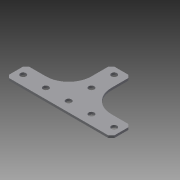
# Autodesk Inventor part: 3x5 T
Saved by Autodesk Inventor 2015 (Build 190159000, 159)
## iProperties
Created: 2015-01-29
Part Number: 3x5 T
Material: Generic
Document SubType Name: Sheet Metal
Designer: chappelled
Density: 1 g/cm^3
Appearance: Default
Sheet Metal Rule: Default
Author: chappelled
Autodesk Inventor part; units mm, degrees
ref_plane "YZ Plane" through (0, 0, 0) normal (1, 0, 0) x (0, 1, 0)
ref_plane "XZ Plane" through (0, 0, 0) normal (0, 1, 0) x (-1, 0, 0)
ref_plane "XY Plane" through (0, 0, 0) normal (0, 0, 1) x (1, 0, 0)
sketch "Sketch1" plane through (0, 0, 0) normal (0, 1, 0) x (-1, 0, 0)
  line L0 (-3.175, 0) -> (-19.05, 0)
  line L1 (-69.85, 50.8) -> (-69.85, 66.675)
  line L2 (-66.675, 69.85) -> (44.45, 69.85)
  line L3 (-66.675, 69.85) -> (-69.85, 66.675)
  line L4 (-22.225, 3.175) -> (-22.225, 22.225)
  line L5 (-47.625, 47.625) -> (-66.675, 47.625)
  arc A0 (-22.225, 22.225) -> (-47.625, 47.625) centre (-47.625, 22.225) ccw
  line L6 (-22.225, 3.175) -> (-19.05, 0)
  line L7 (-69.85, 50.8) -> (-66.675, 47.625)
  line L8 (0, 3.175) -> (0, 22.225)
  line L9 (25.4, 47.625) -> (44.45, 47.625)
  line L10 (47.625, 50.8) -> (47.625, 66.675)
  arc A1 (25.4, 47.625) -> (0, 22.225) centre (25.4, 22.225) ccw
  line L11 (44.45, 69.85) -> (47.625, 66.675)
  line L12 (44.45, 47.625) -> (47.625, 50.8)
  line L13 (-3.175, 0) -> (0, 3.175)
  point P0 (0, 0)
  point P1 (-69.85, 69.85)
  point P2 (-3.175, 0)
  point P3 (0, 0)
  point P4 (-22.225, 47.625)
  point P5 (-22.225, 0)
  point P6 (-69.85, 47.625)
  point P7 (52.01, 70.1655)
  point P8 (52.01, 44.7655)
  point P9 (5.867, 46.0375)
  point P10 (5.867, 11.0567)
  point P11 (0, 47.625)
  point P12 (41.275, 47.625)
  point P13 (47.625, 44.45)
  point P14 (47.625, 63.5)
  point P15 (47.625, 69.85)
  point P16 (47.625, 47.625)
  point P17 (0, 0)
  dimension "d6" = 3.175
  dimension "d7" = 3.175
  dimension "d10" = 25.4
  dimension "d11" = 3.175
  dimension "d12" = 3.175
  dimension "d13" = 3.175
  dimension "d14" = 3.175
  dimension "d39" = 19.05
  dimension "d40" = 19.05
  dimension "d44" = 22.225
  dimension "d45" = 25.4
  dimension "d46" = 3.175
  dimension "d47" = 3.175
  dimension "d48" = 3.175
  dimension "d49" = 3.175
  dimension "d50" = 19.05
  dimension "d56" = 22.225
  dimension "d57" = 22.225
  dimension "d58" = 3.175
  dimension "d59" = 3.175
  constraints: 28 end point, 22 point on line, 4 perpendicular, 4 point on circle, 4 tangent, 2 centre point, 2 parallel, 1 horizontal
  measures "d6" distance of L2.start point (-69.85, 69.85)
  measures "d7" distance of L1.end point (-69.85, 69.85)
  measures "d10" radius of A0
  measures "d11" distance of L4.start point (-22.225, 0)
  measures "d12" distance of L0.end point (-22.225, 0)
  measures "d13" distance of L1.start point (-69.85, 47.625)
  measures "d14" distance of L5.end point (-69.85, 47.625)
  measures "d39" distance of L4.start L4.end
  measures "d40" distance of L5.start L5.end
  measures "d44" distance from line of L2 point (41.275, 47.625)
  measures "d45" radius of A1
  measures "d46" distance of L2.end point (47.625, 69.85)
  measures "d47" distance of L10.end point (47.625, 69.85)
  measures "d48" distance of L9.end point (47.625, 47.625)
  measures "d49" distance of L10.start point (47.625, 47.625)
  measures "d50" distance of L9.start L9.end
  measures "d56" distance between parallel lines of L8 L4
  measures "d57" distance between parallel lines of L2 L5
  measures "d58" distance of L0.start point (0, 0)
  measures "d59" distance of L8.start point (0, 0)
extrude "Extrusion1" add sketch "Sketch1" along normal blind 2.54
hole "Hole1" at (11.1125, 2.54, 58.7375) direction (0, -1, 0) diameter 6.35 end through all
pattern_linear "Rectangular Pattern1" count 5 spacing 25.4 along (1, 0, 0) of "Hole1" first direction both ways yes
pattern_linear "Rectangular Pattern2" count 3 spacing 25.4 along (0, 0, -1) of "Hole1"
equation "\"d6\" = d2"
equation "\"d7\" = d6"
equation "\"d12\" = d11"
equation "\"d13\" = d11"
equation "\"d14\" = d13"
equation "\"d39\" = d50"
equation "\"d40\" = d50"
equation "\"d47\" = d46"
equation "\"d48\" = d46"
equation "\"d49\" = d48"
equation "\"d57\" = d44"
equation "\"d59\" = d58"
equation "\"BendRadius\" = Thickness"
equation "\"BendReliefWidth\" = Thickness"
equation "\"BendReliefDepth\" = 0.5 * Thickness"
equation "\"CornerReliefSize\" = 4 * Thickness"
equation "\"MinimumRemnant\" = 2 * Thickness"
equation "\"TransitionRadius\" = BendRadius"
equation "\"JacobiRadiusSize\" = Thickness"
equation "\"GapSize\" = Thickness"
equation "\"Thickness\" = 3.048"
equation "\"d2\" = 3.175"
body "Solid1"
